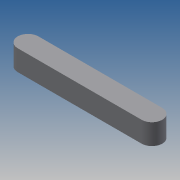
# Autodesk Inventor part: arm
Saved by Autodesk Inventor 2013 (Build 170138000, 138)
## iProperties
Created: 2017-03-06
Part Number: arm
Material: Generic
Document SubType Name: Modeling
Designer: employee
Density: 1 g/cm^3
Author: employee
Autodesk Inventor part; units mm, degrees
ref_plane "YZ Plane" through (0, 0, 0) normal (1, 0, 0) x (0, 1, 0)
ref_plane "XZ Plane" through (0, 0, 0) normal (0, 1, 0) x (-1, 0, 0)
ref_plane "XY Plane" through (0, 0, 0) normal (0, 0, 1) x (1, 0, 0)
sketch "Sketch1" plane through (0, 0, 0) normal (0, 0, 1) x (1, 0, 0)
  line L0 (0, 12.5) -> (150, 12.5)
  arc A0 (150, -12.5) -> (150, 12.5) centre (150, 0) ccw
  line L1 (150, -12.5) -> (0, -12.5)
  arc A1 (0, 12.5) -> (0, -12.5) centre (0, 0) ccw
  dimension "d0" = 150
  dimension "d2" = 12.5
  constraints: 4 end point, 4 point on circle, 4 tangent, 2 centre point, 2 horizontal, 1 coincident
  measures "d0" distance of L0.start L0.end
  measures "d2" radius of A1
extrude "Extrusion1" add sketch "Sketch1" along normal blind 25
body "Solid1"
